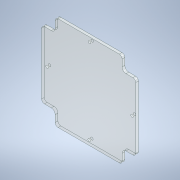
# Autodesk Inventor part: AcrylicPlateForFixturePlate
Saved by Autodesk Inventor 2021 (Build 250183000, 183)
## iProperties
Created: 2020-07-23
Part Number: AcrylicPlateForFixturePlate
Material: Generic
Document SubType Name: Modeling
Designer: CASE-SMALL2
Density: 1 g/cm^3
Appearance: Default
Author: CASE-SMALL2
## iProperties of the stored document _3DPrint.ipt
Created: 2020-07-24
Part Number: _3DPrint
Material: Generic
Document SubType Name: Modeling
Designer: CASE-SMALL2
Density: 1 g/cm^3
Appearance: Default
Author: CASE-SMALL2
Autodesk Inventor part; units mm, degrees
ref_plane "YZ Plane" through (0, 0, 0) normal (1, 0, 0) x (0, 1, 0)
ref_plane "XZ Plane" through (0, 0, 0) normal (0, 1, 0) x (-1, 0, 0)
ref_plane "Work Plane1" through (1.0182, 4.3839, -28.4508) normal (0, 0, 1) x (1, 0, 0)
sketch "Sketch4" plane through (1.0182, 4.3839, -28.4508) normal (0, 0, 1) x (1, 0, 0)
  arc A0 (100, 130) -> (90, 140) centre (90, 130) ccw construction
  line L0 (-90, 140) -> (90, 140) construction
  arc A1 (-90, 140) -> (-100, 130) centre (-90, 130) ccw construction
  line L1 (-100, 110) -> (-100, 130) construction
  arc A2 (-110, 100) -> (-100, 110) centre (-110, 110) ccw construction
  line L2 (-130, 100) -> (-110, 100) construction
  arc A3 (-130, 100) -> (-140, 90) centre (-130, 90) ccw construction
  line L3 (-140, -90) -> (-140, 90) construction
  arc A4 (-140, -90) -> (-130, -100) centre (-130, -90) ccw construction
  line L4 (-110, -100) -> (-130, -100) construction
  arc A5 (-100, -110) -> (-110, -100) centre (-110, -110) ccw construction
  line L5 (-100, -130) -> (-100, -110) construction
  arc A6 (-100, -130) -> (-90, -140) centre (-90, -130) ccw construction
  line L6 (90, -140) -> (-90, -140) construction
  arc A7 (90, -140) -> (100, -130) centre (90, -130) ccw construction
  line L7 (100, -110) -> (100, -130) construction
  arc A8 (110, -100) -> (100, -110) centre (110, -110) ccw construction
  line L8 (130, -100) -> (110, -100) construction
  arc A9 (130, -100) -> (140, -90) centre (130, -90) ccw construction
  line L9 (140, 90) -> (140, -90) construction
  arc A10 (140, 90) -> (130, 100) centre (130, 90) ccw construction
  line L10 (110, 100) -> (130, 100) construction
  arc A11 (100, 110) -> (110, 100) centre (110, 110) ccw construction
  line L11 (100, 130) -> (100, 110) construction
  circle A12 centre (0, 125) radius 3.75 construction
  circle A13 centre (0, -125) radius 3.75 construction
  circle A14 centre (-125, 0) radius 3.75 construction
  circle A15 centre (125, 0) radius 3.75 construction
  arc A16 (98.5, 130) -> (90, 138.5) centre (90, 130) ccw
  line L12 (98.5, 130) -> (98.5, 110)
  arc A17 (98.5, 110) -> (110, 98.5) centre (110, 110) ccw
  line L13 (110, 98.5) -> (130, 98.5)
  arc A18 (138.5, 90) -> (130, 98.5) centre (130, 90) ccw
  line L14 (138.5, 90) -> (138.5, -90)
  arc A19 (130, -98.5) -> (138.5, -90) centre (130, -90) ccw
  line L15 (130, -98.5) -> (110, -98.5)
  arc A20 (110, -98.5) -> (98.5, -110) centre (110, -110) ccw
  line L16 (98.5, -110) -> (98.5, -130)
  arc A21 (90, -138.5) -> (98.5, -130) centre (90, -130) ccw
  line L17 (90, -138.5) -> (-90, -138.5)
  arc A22 (-98.5, -130) -> (-90, -138.5) centre (-90, -130) ccw
  line L18 (-98.5, -130) -> (-98.5, -110)
  arc A23 (-98.5, -110) -> (-110, -98.5) centre (-110, -110) ccw
  line L19 (-110, -98.5) -> (-130, -98.5)
  arc A24 (-138.5, -90) -> (-130, -98.5) centre (-130, -90) ccw
  line L20 (-138.5, -90) -> (-138.5, 90)
  arc A25 (-130, 98.5) -> (-138.5, 90) centre (-130, 90) ccw
  line L21 (-130, 98.5) -> (-110, 98.5)
  arc A26 (-110, 98.5) -> (-98.5, 110) centre (-110, 110) ccw
  line L22 (-98.5, 110) -> (-98.5, 130)
  arc A27 (-90, 138.5) -> (-98.5, 130) centre (-90, 130) ccw
  line L23 (-90, 138.5) -> (90, 138.5)
  line L24 (-125, 0) -> (-113.2017, 0)
  circle A28 centre (2.5, 125) radius 3.75
  circle A29 centre (-122.5, 0) radius 3.75
  circle A30 centre (127.5, 0) radius 3.75
  circle A31 centre (1.5, -125) radius 3.75
  point P0 (-1.0182, -4.3839)
  dimension "d21" = 1.5
  dimension "d22" = 2.5
  dimension "d23" = 2.5
  dimension "d24" = 2.5
  dimension "d25" = 1.5
  dimension "d26" = 7.5
  dimension "d27" = 7.5
  dimension "d28" = 7.5
  dimension "d29" = 7.5
  dimension "d30" = 7.5
  constraints: 26 end point, 24 point on circle, 16 centre point, 1 horizontal, 1 point on line, 23 other
  measures "d21" distance between parallel lines of L0 L23
  measures "d22" distance of L24.start A29.centre
  measures "d23" distance of A12.centre A28.centre
  measures "d24" distance of A30.centre A15.centre
  measures "d25" distance of A13.centre A31.centre
  measures "d26" diameter of A13
  measures "d27" diameter of A31
  measures "d28" diameter of A29
  measures "d29" diameter of A28
  measures "d30" diameter of A30
extrude "Extrusion3" add sketch "Sketch4" along normal blind 8
sketch "Sketch6" plane through (1.0182, 4.3839, -20.4508) normal (0, 0, 1) x (1, 0, 0)
  arc A0 (98.5, 130) -> (90, 138.5) centre (90, 130) ccw projected
  line L0 (90, 138.5) -> (-90, 138.5) projected
  arc A1 (-90, 138.5) -> (-98.5, 130) centre (-90, 130) ccw projected
  line L1 (-98.5, 130) -> (-98.5, 110) projected
  arc A2 (-110, 98.5) -> (-98.5, 110) centre (-110, 110) ccw projected
  line L2 (-110, 98.5) -> (-130, 98.5) projected
  arc A3 (-130, 98.5) -> (-138.5, 90) centre (-130, 90) ccw projected
  line L3 (-138.5, 90) -> (-138.5, -90) projected
  arc A4 (-138.5, -90) -> (-130, -98.5) centre (-130, -90) ccw projected
  line L4 (-130, -98.5) -> (-110, -98.5) projected
  arc A5 (-98.5, -110) -> (-110, -98.5) centre (-110, -110) ccw projected
  line L5 (-98.5, -110) -> (-98.5, -130) projected
  arc A6 (-98.5, -130) -> (-90, -138.5) centre (-90, -130) ccw projected
  line L6 (-90, -138.5) -> (90, -138.5) projected
  arc A7 (90, -138.5) -> (98.5, -130) centre (90, -130) ccw projected
  line L7 (98.5, -130) -> (98.5, -110) projected
  arc A8 (110, -98.5) -> (98.5, -110) centre (110, -110) ccw projected
  line L8 (110, -98.5) -> (130, -98.5) projected
  arc A9 (130, -98.5) -> (138.5, -90) centre (130, -90) ccw projected
  line L9 (138.5, -90) -> (138.5, 90) projected
  arc A10 (138.5, 90) -> (130, 98.5) centre (130, 90) ccw projected
  line L10 (130, 98.5) -> (110, 98.5) projected
  arc A11 (98.5, 110) -> (110, 98.5) centre (110, 110) ccw projected
  line L11 (98.5, 110) -> (98.5, 130) projected
  circle A12 centre (1.5, -125) radius 3.75 projected
  circle A13 centre (127.5, 0) radius 3.75 projected
  circle A14 centre (-122.5, 0) radius 3.75 projected
  circle A15 centre (2.5, 125) radius 3.75 projected
  point P0 (-1.0182, -4.3839)
equation "\"d27\" = d26"
equation "\"d28\" = d27"
equation "\"d29\" = d28"
equation "\"d30\" = d28"
body "Solid2"
